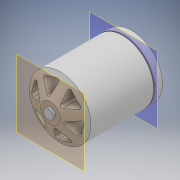
# Autodesk Inventor part: motor
Saved by Autodesk Inventor 2018 (Build 220112000, 112)
## iProperties
Created: 2017-06-05
Part Number: motor
Material: Generic
Document SubType Name: Modeling
Designer: Zadeka
Density: 1 g/cm^3
Appearance: Default
Author: Zadeka
Autodesk Inventor part; units mm, degrees
ref_plane "YZ Plane" through (0, 0, 0) normal (1, 0, 0) x (0, 1, 0)
ref_plane "XZ Plane" through (0, 0, 0) normal (0, 1, 0) x (-1, 0, 0)
ref_plane "XY Plane" through (0, 0, 0) normal (0, 0, 1) x (1, 0, 0)
sketch "Sketch1" plane through (0, 0, 0) normal (0, 1, 0) x (-1, 0, 0)
  circle A0 centre (0, 0) radius 31.5
  dimension "d0" = 63
  constraints: 1 centre point, 1 coincident
  measures "d0" diameter of A0
extrude "Extrusion1" add sketch "Sketch1" along normal blind 64
ref_plane "Work Plane1" through (0, -10, 0) normal (0, -1, 0) x (1, 0, 0)
sketch "Sketch2" plane through (0, -10, 0) normal (0, -1, 0) x (1, 0, 0)
  circle A0 centre (0, 0) radius 10
  dimension "d4" = 20
  constraints: 1 centre point, 1 coincident
  measures "d4" diameter of A0
loft "Loft1" add profiles "Sketch2" section 1 edges at (31.5, 0, 0)
sketch "Sketch3" plane through (0, -10, 0) normal (0, -1, 0) x (1, 0, 0)
  circle A0 centre (0, 0) radius 5
  dimension "d9" = 10
  constraints: 1 centre point, 1 coincident
  measures "d9" diameter of A0
extrude "Extrusion2" add sketch "Sketch3" along normal blind 2
ref_plane "Work Plane2" through (0, 65, 0) normal (0, 1, 0) x (1, 0, 0)
sketch "Sketch4" plane through (0, 65, 0) normal (0, 1, 0) x (1, 0, 0)
  circle A0 centre (0, 0) radius 31.5
  dimension "d13" = 63
  constraints: 1 centre point, 1 coincident
  measures "d13" diameter of A0
extrude "Extrusion3" add sketch "Sketch4" along normal blind 8
sketch "Sketch5" plane through (0, -10, 0) normal (0, -1, 0) x (1, 0, 0)
  point P0 (0, 0)
sketch "Sketch6" plane through (0, -10, 0) normal (0, -1, 0) x (1, 0, 0)
  line L0 (0, 0) -> (0, -31.5)
  circle A0 centre (0, 0) radius 31.5 projected
  line L1 (0, 0) -> (-31.5, 0)
  line L2 (-15.75, 0) -> (0, -15.75)
  line L3 (-7.875, -7.875) -> (-18.4816, -18.4816)
  line L4 (-18.4816, -18.4816) -> (-22.9102, -14.053)
  line L5 (-18.4816, -18.4816) -> (-14.053, -22.9102)
  line L6 (-21.8882, -10.6776) -> (-10.8167, -8.4633)
  line L7 (-10.6776, -21.8882) -> (-8.4633, -10.8167)
  arc A1 (-21.8882, -10.6776) -> (-22.9102, -14.053) centre (-21.496, -12.6388) ccw
  arc A2 (-8.4633, -10.8167) -> (-10.8167, -8.4633) centre (-10.4245, -10.4245) ccw
  arc A3 (-14.053, -22.9102) -> (-10.6776, -21.8882) centre (-12.6388, -21.496) ccw
  line L8 (-1.697, -24.2946) -> (1.9211, -13.5992)
  arc A4 (-1.697, -24.2946) -> (0.7152, -26.8673) centre (0.1975, -24.9355) ccw
  line L9 (6.7647, -25.2463) -> (0.7152, -26.8673)
  line L10 (6.7647, -25.2463) -> (12.8143, -23.6254)
  arc A5 (12.8143, -23.6254) -> (13.6169, -20.1912) centre (12.2967, -21.6935) ccw
  line L11 (13.6169, -20.1912) -> (5.1359, -12.7378)
  arc A6 (5.1359, -12.7378) -> (1.9211, -13.5992) centre (3.8156, -14.2401) ccw
  line L12 (20.1912, -13.6169) -> (12.7378, -5.1359)
  arc A7 (20.1912, -13.6169) -> (23.6254, -12.8143) centre (21.6935, -12.2967) ccw
  line L13 (25.2463, -6.7647) -> (23.6254, -12.8143)
  line L14 (25.2463, -6.7647) -> (26.8673, -0.7152)
  arc A8 (26.8673, -0.7152) -> (24.2946, 1.697) centre (24.9355, -0.1975) ccw
  line L15 (24.2946, 1.697) -> (13.5992, -1.9211)
  arc A9 (13.5992, -1.9211) -> (12.7378, -5.1359) centre (14.2401, -3.8156) ccw
  line L16 (21.8882, 10.6776) -> (10.8167, 8.4633)
  arc A10 (21.8882, 10.6776) -> (22.9102, 14.053) centre (21.496, 12.6388) ccw
  line L17 (18.4816, 18.4816) -> (22.9102, 14.053)
  line L18 (18.4816, 18.4816) -> (14.053, 22.9102)
  arc A11 (14.053, 22.9102) -> (10.6776, 21.8882) centre (12.6388, 21.496) ccw
  line L19 (10.6776, 21.8882) -> (8.4633, 10.8167)
  arc A12 (8.4633, 10.8167) -> (10.8167, 8.4633) centre (10.4245, 10.4245) ccw
  line L20 (1.697, 24.2946) -> (-1.9211, 13.5992)
  arc A13 (1.697, 24.2946) -> (-0.7152, 26.8673) centre (-0.1975, 24.9355) ccw
  line L21 (-6.7647, 25.2463) -> (-0.7152, 26.8673)
  line L22 (-6.7647, 25.2463) -> (-12.8143, 23.6254)
  arc A14 (-12.8143, 23.6254) -> (-13.6169, 20.1912) centre (-12.2967, 21.6935) ccw
  line L23 (-13.6169, 20.1912) -> (-5.1359, 12.7378)
  arc A15 (-5.1359, 12.7378) -> (-1.9211, 13.5992) centre (-3.8156, 14.2401) ccw
  line L24 (-20.1912, 13.6169) -> (-12.7378, 5.1359)
  arc A16 (-20.1912, 13.6169) -> (-23.6254, 12.8143) centre (-21.6935, 12.2967) ccw
  line L25 (-25.2463, 6.7647) -> (-23.6254, 12.8143)
  line L26 (-25.2463, 6.7647) -> (-26.8673, 0.7152)
  arc A17 (-26.8673, 0.7152) -> (-24.2946, -1.697) centre (-24.9355, 0.1975) ccw
  line L27 (-24.2946, -1.697) -> (-13.5992, 1.9211)
  arc A18 (-13.5992, 1.9211) -> (-12.7378, 5.1359) centre (-14.2401, 3.8156) ccw
  point P0 (-25.5527, -11.4105)
  point P1 (-11.4105, -25.5527)
  point P2 (-2.8945, -27.8345)
  point P3 (2.8825, -10.7575)
  point P4 (16.424, -22.6581)
  point P5 (22.6581, -16.424)
  point P6 (10.7575, -2.8825)
  point P7 (27.8345, 2.8945)
  point P8 (25.5527, 11.4105)
  point P9 (7.875, 7.875)
  point P10 (11.4105, 25.5527)
  point P11 (2.8945, 27.8345)
  point P12 (-2.8825, 10.7575)
  point P13 (-16.424, 22.6581)
  point P14 (-22.6581, 16.424)
  point P15 (-10.7575, 2.8825)
  point P16 (-27.8345, -2.8945)
  dimension "d16" = 15
  dimension "d17" = 10
  dimension "d18" = 10
  dimension "d19" = 2
  dimension "d22" = 360
  constraints: 56 end point, 38 point on circle, 36 point on line, 18 centre point, 6 tangent, 3 midpoint, 2 equal radius, 2 perpendicular, 1 vertical, 121 other
  measures "d16" distance of L3.start L3.end
  measures "d17" distance of L3.end point (-25.553, -11.411)
  measures "d18" distance of L3.end point (-11.411, -25.553)
  measures "d19" radius of A1
extrude "Extrusion4" cut sketch "Sketch6" against normal blind 70.25 contours L8 A6 L11 A5 L10 L9 A4 L0 | L0 A4 L8 | L27 A17 L1 | L1 A17 L26 L25 A16 L24 A18 L27 | A2 L7 A3 L5 L3 | L3 L4 A1 L6 A2 | L12 A9 L15 A8 L14 L13 A7 | L16 A12 L19 A11 L18 L17 A10 | L20 A15 L23 A14 L22 L21 A13
body "Solid1"
